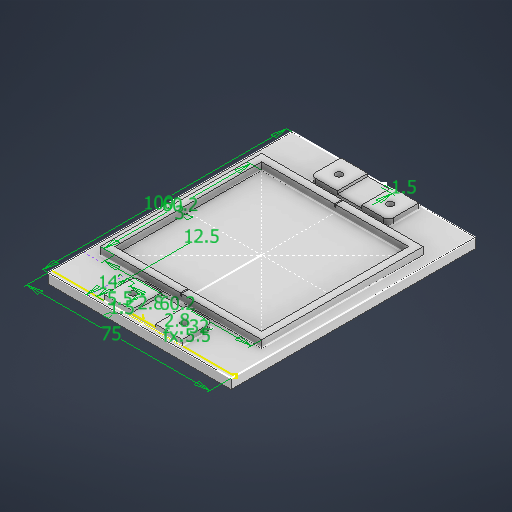
# Autodesk Inventor part: Molde 663FBR 1mm
Saved by Autodesk Inventor 2026.1 (Build 301233000, 233)
## iProperties
Created: 2025-07-30
Part Number: Molde 663FBR 1mm
Material: Genérico
Document SubType Name: Modeling
Designer: Laboratorio_sensores
Density: 1 g/cm^3
Appearance: Valor por defecto
Author: Laboratorio_sensores
Autodesk Inventor part; units mm, degrees
ref_plane "YZ Plane" through (0, 0, 0) normal (1, 0, 0) x (0, 1, 0)
ref_plane "XZ Plane" through (0, 0, 0) normal (0, 1, 0) x (-1, 0, 0)
ref_plane "XY Plane" through (0, 0, 0) normal (0, 0, 1) x (1, 0, 0)
sketch "Boceto1" plane through (0, 0, 0) normal (0, 1, 0) x (-1, 0, 0)
  line L0 (0, 0) -> (75, 0)
  line L1 (75, 0) -> (75, -100)
  line L2 (75, -100) -> (0, -100)
  line L3 (0, -100) -> (0, 0)
  line L4 (7.4, -80.1) -> (67.6, -80.1)
  line L5 (67.6, -80.1) -> (67.6, -19.9)
  line L6 (67.6, -19.9) -> (7.4, -19.9)
  line L7 (7.4, -19.9) -> (7.4, -80.1)
  line L8 (7.4, -80.1) -> (67.6, -19.9) construction
  line L9 (67.6, -80.1) -> (7.4, -19.9) construction
  line L10 (70.6, -16.9) -> (70.6, -83.1)
  line L11 (70.6, -83.1) -> (4.4, -83.1)
  line L12 (4.4, -83.1) -> (4.4, -16.9)
  line L13 (4.4, -16.9) -> (70.6, -16.9)
  line L14 (53.5, -1.5) -> (21.5, -1.5)
  line L15 (21.5, -1.5) -> (21.5, -14)
  line L16 (21.5, -14) -> (53.5, -14)
  line L17 (53.5, -14) -> (53.5, -1.5)
  line L18 (67.6, -50) -> (7.4, -50) construction
  line L19 (53.5, -7.75) -> (48, -7.75) construction
  line L20 (48, -7.75) -> (27, -7.75) construction
  line L21 (27, -7.75) -> (21.5, -7.75) construction
  circle A0 centre (48, -7.75) radius 1.4
  circle A1 centre (27, -7.75) radius 1.4
  line L22 (53.5, -98.5) -> (21.5, -98.5)
  line L23 (21.5, -98.5) -> (21.5, -86)
  line L24 (21.5, -86) -> (53.5, -86)
  line L25 (53.5, -86) -> (53.5, -98.5)
  circle A2 centre (48, -92.25) radius 1.4
  circle A3 centre (27, -92.25) radius 1.4
  line L26 (58.4347, 0) -> (58.4347, -14) construction
  line L27 (68.2, -14.5) -> (75, -14.5) construction
  line L28 (37.5, -19.9) -> (37.5, -80.1) construction
  circle A4 centre (48, -92.25) radius 1.4
  line L29 (48, -7.75) -> (27, -7.75)
  line L30 (37.5, -1.5) -> (37.5, 0)
  line L31 (37.5, -1.5) -> (37.5, -50)
  point P0 (37.5, -14)
  point P1 (37.5, -16.9)
  point P2 (37.5, -98.5)
  point P3 (37.5, -100)
  dimension "d0" = 100
  dimension "d1" = 75
  dimension "d2" = 60.2
  dimension "d3" = 60.2
  dimension "d4" = 3
  dimension "d5" = 12.5
  dimension "d6" = 32
  dimension "d8" = 5.5
  dimension "d9" = 5.5
  dimension "d10" = 2.8
  dimension "d11" = 2.8
  dimension "d14" = 14
  dimension "d32" = 1.5
  dimension "d36" = 1.5
  constraints: 64 end point, 14 midpoint, 8 parallel, 7 symmetric about line, 6 perpendicular, 5 centre point, 4 horizontal, 3 point on line, 2 coincident, 2 collinear, 1 vertical, 6 other
  measures "d0" distance of L0.end L1.end
  measures "d1" distance of L0.start L0.end
  measures "d2" distance of L4.end L5.end
  measures "d3" distance of L5.end L6.end
  measures "d4" distance between parallel lines of L5 L10
  measures "d5" distance of L16.end L14.start
  measures "d6" distance of L15.end L16.end
  measures "d8" distance of L19.start L19.end
  measures "d9" distance of L20.end L21.end
  measures "d10" diameter of A0
  measures "d11" diameter of A1
  measures "d14" distance of L26.start L26.end
  measures "d32" distance between parallel lines of L0 L14
  measures "d36" distance of point (37.5, -98.5) point (37.5, -100)
extrude "Extrusión1" add sketch "Boceto1" along normal blind 3 contours L10 L11 L12 L13
extrude "Extrusión2" add sketch "Boceto1" against normal blind 4 contours L0 L1 L2 L3 | L17 L16 L31 L14 | L31 L16 L15 L14 | L22 L23 L24 L25
extrude "Extrusión3" add sketch "Boceto1" along normal blind 2.25 contours L17 L16 L31 L14 | L31 L16 L15 L14 | L22 L23 L24 L25
sketch "Boceto2" plane through (0, 2.25, 0) normal (0, 1, 0) x (1, 0, 0)
  line L0 (-53.5, 1.5) -> (-21.5, 1.5) projected
  line L1 (-37.5, 1.5) -> (-37.5, 14)
  line L2 (-21.5, 14) -> (-53.5, 14) projected
  line L3 (-32.5, 1.5) -> (-42.5, 1.5)
  line L4 (-42.5, 1.5) -> (-42.5, 14)
  line L5 (-42.5, 14) -> (-32.5, 14)
  line L6 (-32.5, 14) -> (-32.5, 1.5)
  line L7 (-32.5, 1.5) -> (-42.5, 14) construction
  line L8 (-42.5, 1.5) -> (-32.5, 14) construction
  line L9 (-67.6, 50) -> (-7.4, 50) construction
  line L10 (-53.5, 98.5) -> (-21.5, 98.5)
  line L11 (-21.5, 86) -> (-53.5, 86)
  line L12 (-42.5, 98.5) -> (-42.5, 86)
  line L13 (-32.5, 86) -> (-32.5, 98.5)
  point P0 (0, 0)
  point P1 (-37.5, 7.75)
  point P2 (-42.5, 98.5)
  point P3 (-42.5, 1.5)
  point P4 (-32.5, 1.5)
  point P5 (-32.5, 14)
  dimension "d22" = 10
  constraints: 22 end point, 8 symmetric about line, 5 midpoint, 2 parallel, 2 point on line, 1 horizontal, 1 perpendicular
  measures "d22" distance between parallel lines of L4 L6
extrude "Extrusión4" cut sketch "Boceto2" against normal blind 1.1
extrude "Extrusión5" add sketch "Boceto1" against normal blind 4 contours L7 L6 L5 L4 | L10 L11 L12 L13
sketch "Boceto3" plane through (0, 3, 0) normal (0, 1, 0) x (1, 0, 0)
  line L0 (-37.5, 19.9) -> (-37.5, 80.1) construction
  line L1 (-70.6, 16.9) -> (-4.4, 16.9) projected
  line L2 (-37.5, 16.9) -> (-37.5, 83.1)
  line L3 (-4.4, 83.1) -> (-70.6, 83.1) projected
  line L4 (-37.25, 16.9) -> (-37.75, 16.9)
  line L5 (-37.75, 16.9) -> (-37.75, 83.1)
  line L6 (-37.75, 83.1) -> (-37.25, 83.1)
  line L7 (-37.25, 83.1) -> (-37.25, 16.9)
  line L8 (-37.25, 16.9) -> (-37.75, 83.1) construction
  line L9 (-37.75, 16.9) -> (-37.25, 83.1) construction
  point P0 (0, 0)
  point P1 (-37.5, 50)
  point P2 (-37.25, 16.9)
  point P3 (-37.25, 83.1)
  point P4 (-37.75, 16.9)
  dimension "d27" = 0.5
  constraints: 14 end point, 5 midpoint, 2 parallel, 1 horizontal, 1 perpendicular, 1 point on line
  measures "d27" distance between parallel lines of L5 L7
extrude "Extrusión6" cut sketch "Boceto3" against normal blind 1
sketch "Boceto4" plane through (-53.5, 0, -1.5) normal (0, 0, 1) x (1, 0, 0)
  line L0 (16.25, 2) -> (15.75, 2) projected
  line L1 (21, 1.15) -> (11, 1.15) projected
  line L2 (-21.5, 0) -> (53.5, 0) projected
  line L3 (15.75, 2) -> (15.75, 3) projected
fillet "Empalme1" radius 2 4 edges at (-53.5, 1.125, -86) (-21.5, 1.125, -86) (-21.5, 1.125, -14) (-53.5, 1.125, -14)
sketch "Boceto5" plane through (-53.5, 0, -1.5) normal (0, 0, 1) x (1, 0, 0)
  line L0 (16.25, 2) -> (15.75, 2) projected
  line L1 (21, 1.15) -> (11, 1.15) projected
  point P0 (53.5, 0)
equation "\"d9\" = d8"
